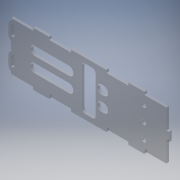
# Autodesk Inventor part: Top_plate2
Saved by Autodesk Inventor 2016 (Build 200138000, 138)
## iProperties
Created: 2015-06-18
Part Number: Top_plate2
Material: Generic
Document SubType Name: Modeling
Designer: Openlab
Density: 1 g/cm^3
Appearance: Polycarbonate - Clear
Author: Openlab
Autodesk Inventor part; units mm, degrees
ref_plane "YZ Plane" through (0, 0, 0) normal (1, 0, 0) x (0, 1, 0)
ref_plane "XZ Plane" through (0, 0, 0) normal (0, 1, 0) x (-1, 0, 0)
ref_plane "XY Plane" through (0, 0, 0) normal (0, 0, 1) x (1, 0, 0)
sketch "Sketch1" plane through (0, 0, 0) normal (0, 1, 0) x (-1, 0, 0)
  line L0 (37.25, -2.25) -> (24.75, -2.25) construction
  line L1 (24.75, -2.25) -> (24.75, -14.75) construction
  line L2 (24.75, -14.75) -> (37.25, -14.75) construction
  line L3 (37.25, -14.75) -> (37.25, -2.25) construction
  line L4 (56.9183, -8.5) -> (8.3915, -8.5) construction
  line L5 (0, -17) -> (105, -17) construction
  line L6 (0, 0) -> (0, -51) construction
  line L7 (0, -34) -> (105, -34) construction
  line L8 (105, -51) -> (105, 0) construction
  line L9 (31, 19) -> (31, -51) construction
  line L10 (56.8064, -25.5) -> (17, -25.5) construction
  line L11 (24.75, -19.25) -> (24.75, -31.75) construction
  line L12 (37.25, -19.25) -> (24.75, -19.25) construction
  line L13 (37.25, -31.75) -> (37.25, -19.25) construction
  line L14 (24.75, -31.75) -> (37.25, -31.75) construction
  line L15 (24.75, -36.25) -> (24.75, -48.75) construction
  line L16 (37.25, -36.25) -> (24.75, -36.25) construction
  line L17 (37.25, -48.75) -> (37.25, -36.25) construction
  line L18 (24.75, -48.75) -> (37.25, -48.75) construction
  line L19 (56.3008, -42.5) -> (16.5498, -42.5) construction
  arc A0 (53.45, -12) -> (53.45, -22) centre (53.45, -17) ccw
  arc A1 (92, -22) -> (92, -12) centre (92, -17) ccw
  arc A2 (53.45, -29) -> (53.45, -39) centre (53.45, -34) ccw
  arc A3 (92, -39) -> (92, -29) centre (92, -34) ccw
  line L20 (53.45, -12) -> (92, -12)
  line L21 (53.45, -22) -> (92, -22)
  line L22 (53.45, -29) -> (92, -29)
  line L23 (53.45, -39) -> (92, -39)
  arc A4 (16.15, -39) -> (16.15, -29) centre (16.15, -34) ccw
  line L24 (103.5, -49.5) -> (103.5, -1.5) construction
  line L25 (1.5, -1.5) -> (1.5, -49.5) construction
  arc A5 (14, -29) -> (14, -39) centre (14, -34) ccw
  arc A6 (14, -12) -> (14, -22) centre (14, -17) ccw
  line L26 (16.15, -39) -> (14, -39)
  line L27 (14, -29) -> (16.15, -29)
  line L28 (14, -22) -> (16.15, -22)
  line L29 (16.15, -12) -> (14, -12)
  arc A7 (16.15, -22) -> (16.15, -12) centre (16.15, -17) ccw
  arc A8 (96.5, -51) -> (93, -47.5) centre (93, -51) ccw construction
  arc A9 (53.45, -47.5) -> (49.95, -51) centre (53.45, -51) ccw construction
  arc A10 (97.7697, -49.5) -> (93, -46) centre (93, -51) ccw construction
  line L30 (93, -46) -> (53.45, -46) construction
  line L31 (96.5, -51) -> (105, -51) construction
  line L32 (93, -47.5) -> (53.45, -47.5) construction
  line L33 (105, -49.5) -> (97.7697, -49.5) construction
  arc A11 (53.45, -46) -> (48.6803, -49.5) centre (53.45, -51) ccw construction
  arc A12 (48.6803, -1.5) -> (53.45, -5) centre (53.45, 0) ccw construction
  arc A13 (49.95, 0) -> (53.45, -3.5) centre (53.45, 0) ccw construction
  line L34 (93, -3.5) -> (53.45, -3.5) construction
  line L35 (93, -5) -> (53.45, -5) construction
  line L36 (97.7697, -1.5) -> (105, -1.5) construction
  line L37 (105, 0) -> (96.5, 0) construction
  arc A14 (93, -3.5) -> (96.5, 0) centre (93, 0) ccw construction
  arc A15 (93, -5) -> (97.7697, -1.5) centre (93, 0) ccw construction
  arc A16 (16.65, -51) -> (13.15, -47.5) centre (13.15, -51) ccw construction
  arc A17 (12, -47.5) -> (8.5, -51) centre (12, -51) ccw construction
  line L38 (13.15, -46) -> (12, -46) construction
  line L39 (13.15, -47.5) -> (12, -47.5) construction
  arc A18 (12, -46) -> (7.2303, -49.5) centre (12, -51) ccw construction
  arc A19 (17.9197, -49.5) -> (13.15, -46) centre (13.15, -51) ccw construction
  line L40 (48.6803, -49.5) -> (17.9197, -49.5) construction
  line L41 (7.2303, -49.5) -> (0, -49.5) construction
  line L42 (0, -51) -> (8.5, -51) construction
  line L43 (16.65, -51) -> (49.95, -51) construction
  line L44 (13.15, -5) -> (12, -5) construction
  line L45 (13.15, -3.5) -> (12, -3.5) construction
  arc A20 (8.5, 0) -> (12, -3.5) centre (12, 0) ccw construction
  arc A21 (13.15, -3.5) -> (16.65, 0) centre (13.15, 0) ccw construction
  arc A22 (7.2303, -1.5) -> (12, -5) centre (12, 0) ccw construction
  arc A23 (13.15, -5) -> (17.9197, -1.5) centre (13.15, 0) ccw construction
  line L46 (49.95, 0) -> (16.65, 0) construction
  line L47 (8.5, 0) -> (0, 0) construction
  line L48 (0, -1.5) -> (7.2303, -1.5) construction
  line L49 (17.9197, -1.5) -> (48.6803, -1.5) construction
  arc A24 (38.75, -4.25) -> (35.25, -0.75) centre (35.25, -4.25) ccw
  arc A25 (26.75, -0.75) -> (23.25, -4.25) centre (26.75, -4.25) ccw
  arc A26 (35.25, -50.25) -> (38.75, -46.75) centre (35.25, -46.75) ccw
  arc A27 (23.25, -46.75) -> (26.75, -50.25) centre (26.75, -46.75) ccw
  line L50 (38.75, -4.25) -> (38.75, -46.75)
  line L51 (35.25, -0.75) -> (26.75, -0.75)
  line L52 (23.25, -4.25) -> (23.25, -46.75)
  line L53 (26.75, -50.25) -> (35.25, -50.25)
  line L54 (51, -56) -> (51, -53)
  line L55 (11, -56) -> (11, -53)
  line L56 (76, -56) -> (76, -53)
  line L57 (94, -53) -> (94, -56)
  line L58 (-32, -56) -> (-32, -53)
  line L59 (94, 2) -> (94, 5)
  line L60 (76, 2) -> (76, 5)
  line L61 (51, 2) -> (51, 5)
  line L62 (11, 2) -> (11, 5)
  line L63 (-32, 2) -> (-32, 5)
  line L64 (-32, -53) -> (-57, -53)
  line L65 (-14, -53) -> (11, -53)
  line L66 (51, -53) -> (76, -53)
  line L67 (94, -53) -> (119, -53)
  line L68 (119, 2) -> (94, 2)
  line L69 (76, 2) -> (51, 2)
  line L70 (11, 2) -> (-14, 2)
  line L71 (-32, 2) -> (-57, 2)
  line L72 (-14, -53) -> (-14, -56)
  line L73 (-14, 5) -> (-14, 2)
  circle A28 centre (-31.5, -42.5) radius 2.5
  circle A29 centre (-31.5, -25.5) radius 2.5
  circle A30 centre (-31.5, -8.5) radius 2.5
  line L74 (51, 5) -> (11, 5)
  line L75 (94, 5) -> (76, 5)
  line L76 (-14, 5) -> (-32, 5)
  line L77 (94, -56) -> (76, -56)
  line L78 (51, -56) -> (11, -56)
  line L79 (-14, -56) -> (-32, -56)
  line L80 (-57, -20.5) -> (-60, -20.5)
  line L81 (-60, -20.5) -> (-60, -30.5)
  line L82 (-60, -30.5) -> (-57, -30.5)
  line L83 (-57, 2) -> (-57, -20.5)
  line L84 (-57, -30.5) -> (-57, -53)
  line L85 (119, -5.5) -> (116, -5.5)
  line L86 (116, -5.5) -> (116, -15.5)
  line L87 (116, -15.5) -> (119, -15.5)
  line L88 (119, -15.5) -> (119, -5.5)
  line L89 (119, -35.5) -> (116, -35.5)
  line L90 (116, -35.5) -> (116, -45.5)
  line L91 (116, -45.5) -> (119, -45.5)
  line L92 (119, -45.5) -> (119, -35.5)
  arc A31 (119, -20.6962) -> (122, -15.5) centre (116, -15.5) ccw
  line L93 (119, -20.6962) -> (119, -30.3038)
  arc A32 (122, -35.5) -> (119, -30.3038) centre (116, -35.5) ccw
  line L94 (122, -5.5) -> (122, -15.5)
  line L95 (122, -35.5) -> (122, -45.5)
  arc A33 (122, -5.5) -> (119, -0.3038) centre (116, -5.5) ccw
  line L96 (119, -0.3038) -> (119, 2)
  arc A34 (119, -50.6962) -> (122, -45.5) centre (116, -45.5) ccw
  line L97 (119, -50.6962) -> (119, -53)
  point P0 (31, -8.5)
  point P1 (31, -42.5)
  point P2 (31, -25.5)
  dimension "d0" = 12.5
  dimension "d1" = 12.5
  dimension "d2" = 17
  dimension "d3" = 31
  dimension "d4" = 105
  dimension "d5" = 17
  dimension "d6" = 17
  dimension "d7" = 10
  dimension "d8" = 1.5
  dimension "d9" = 1.5
  dimension "d10" = 5
  dimension "d11" = 1.5
  dimension "d12" = 1.5
  dimension "d13" = 1.5
  dimension "d14" = 17
  dimension "d15" = 17
  dimension "d16" = 12
  dimension "d17" = 13
  dimension "d19" = 11.6
  dimension "d20" = 8.6
  dimension "d21" = 12
  dimension "d28" = 2
  dimension "d29" = 2
  dimension "d30" = 7
  dimension "d31" = 2
  dimension "d32" = 2
  dimension "d38" = 40
  dimension "d39" = 25
  dimension "d40" = 18
  dimension "d56" = 3
  dimension "d64" = 14
  dimension "d65" = 22.45
  dimension "d66" = 10.5
  dimension "d67" = 2
  dimension "d109" = 5
  dimension "d118" = 25
  dimension "d120" = 18
  dimension "d127" = 10
  dimension "d128" = 25
  dimension "d129" = 25.5
  dimension "d131" = 10
  dimension "d132" = 3
  dimension "d134" = 20
  dimension "d135" = 28
  dimension "d136" = 3
  constraints: 197 end point, 64 point on circle, 37 collinear, 36 tangent, 35 centre point, 31 point on line, 27 equal radius, 23 perpendicular, 20 parallel, 16 horizontal, 14 coincident, 13 vertical alignment, 9 horizontal alignment, 6 equal length, 6 vertical, 12 other
  measures "d0" distance of L2.end L1.end
  measures "d1" distance of L0.end L1.end
  measures "d2" distance between parallel lines of L10 L4
  measures "d3" distance between parallel lines of L6 L9
  measures "d4" distance between parallel lines of L6 L8
  measures "d5" distance between parallel lines of L19 L10
  measures "d6" distance between parallel lines of L5 L7
  measures "d7" diameter of A0
  measures "d8" distance between parallel lines of L6 L25
  measures "d9" distance between parallel lines of L8 L24
  measures "d10" radius of A4
  measures "d11" radial gap between concentric circles of A8 A10
  measures "d12" distance between parallel lines of L37 L36
  measures "d13" distance between parallel lines of L41 L42
  measures "d14" distance between parallel lines of L7 L42
  measures "d15" distance between parallel lines of L47 L5
  measures "d16" distance from line of A8.centre L8
  measures "d17" distance from line of L8 A3.centre
  measures "d19" distance from line of A19.centre L15
  measures "d20" distance from line of A4.centre L15
  measures "d21" distance from line of L6 A22.centre
  measures "d28" distance from line of L1 A25.centre
  measures "d29" distance from line of A25.centre L0
  measures "d30" diameter of A25
  measures "d31" distance from line of L17 A26.centre
  measures "d32" distance from line of L18 A26.centre
  measures "d38" distance between parallel lines of L55 L54
  measures "d39" distance between parallel lines of L56 L54
  measures "d40" distance between parallel lines of L56 L57
  measures "d56" distance of L60.start L60.end
  measures "d64" distance of L5.start A6.centre
  measures "d65" distance from line of L9 A11.centre
  measures "d66" distance between parallel lines of L65 L19
  measures "d67" distance between parallel lines of L31 L67
  measures "d109" diameter of A28
  measures "d118" distance between parallel lines of L72 L55
  measures "d120" distance of L72.end L58.start
  measures "d127" distance between parallel lines of L82 L80
  measures "d128" distance between parallel lines of L84 L58
  measures "d129" distance from line of L83 A30.centre
  measures "d131" distance of L85.end L86.end
  measures "d132" distance of L85.start L85.end
  measures "d134" distance between parallel lines of L89 L87
  measures "d135" distance between parallel lines of L57 L95
  measures "d136" distance between parallel lines of L95 L92
extrude "Extrusion2" add sketch "Sketch1" along normal blind 3
body "Solid2"
